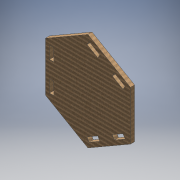
# Autodesk Inventor part: LightDiskTop
Saved by Autodesk Inventor 2016 (Build 200138000, 138)
## iProperties
Created: 2015-12-14
Part Number: LightDiskTop
Material: MDF Medium Density Fiberboard
Document SubType Name: Modeling
Designer: momem
Density: 0.8 g/cm^3
Appearance: Cardboard - Corrugated
Author: momem
Autodesk Inventor part; units mm, degrees
ref_plane "YZ Plane" through (0, 0, 0) normal (1, 0, 0) x (0, 1, 0)
ref_plane "XZ Plane" through (0, 0, 0) normal (0, 1, 0) x (-1, 0, 0)
ref_plane "XY Plane" through (0, 0, 0) normal (0, 0, 1) x (1, 0, 0)
sketch "Sketch1" plane through (0, 0, 0) normal (0, 1, 0) x (-1, 0, 0)
  circle A0 centre (0, 0) radius 30 construction
  line L0 (64.9519, -37.5) -> (0, -75)
  line L1 (0, -75) -> (-64.9519, -37.5)
  line L2 (-64.9519, -37.5) -> (-64.9519, 37.5)
  line L3 (-64.9519, 37.5) -> (0, 75)
  line L4 (0, 75) -> (64.9519, 37.5)
  line L5 (64.9519, 37.5) -> (64.9519, -37.5)
  line L6 (58.5619, 31.7388) -> (52.2358, 31.7388)
  line L7 (52.2358, 31.7388) -> (52.2358, 12.78)
  line L8 (52.2358, 12.78) -> (58.5619, 12.78)
  line L9 (58.5619, 12.78) -> (58.5619, 31.7388)
  line L10 (64.9519, 0) -> (0, 0) construction
  line L11 (58.5619, -31.7388) -> (52.2358, -31.7388)
  line L12 (52.2358, -31.7388) -> (52.2358, -12.78)
  line L13 (52.2358, -12.78) -> (58.5619, -12.78)
  line L14 (58.5619, -12.78) -> (58.5619, -31.7388)
  line L15 (-40.3488, 44.3261) -> (-56.7676, 34.8467)
  line L16 (-56.7676, 34.8467) -> (-53.6045, 29.3681)
  line L17 (-53.6045, 29.3681) -> (-37.1857, 38.8475)
  line L18 (-37.1857, 38.8475) -> (-40.3488, 44.3261)
  line L19 (-15.0501, 51.6275) -> (-18.2131, 57.1061)
  line L20 (-18.2131, 57.1061) -> (-1.7943, 66.5855)
  line L21 (-1.7943, 66.5855) -> (1.3687, 61.1069)
  line L22 (1.3687, 61.1069) -> (-15.0501, 51.6275)
  line L23 (-18.2131, -57.1061) -> (-1.7943, -66.5855)
  line L24 (-1.7943, -66.5855) -> (1.3687, -61.1069)
  line L25 (1.3687, -61.1069) -> (-15.0501, -51.6275)
  line L26 (-15.0501, -51.6275) -> (-18.2131, -57.1061)
  line L27 (-37.1857, -38.8475) -> (-40.3488, -44.3261)
  line L28 (-40.3488, -44.3261) -> (-56.7676, -34.8467)
  line L29 (-56.7676, -34.8467) -> (-53.6045, -29.3681)
  line L30 (-53.6045, -29.3681) -> (-37.1857, -38.8475)
  dimension "d0" = 60
  dimension "d2" = 150
  dimension "d3" = 6.3261
  dimension "d4" = 18.9588
  dimension "d5" = 6.39
  dimension "d6" = 12.78
  dimension "d9" = 360
  constraints: 62 end point, 4 symmetric about line, 2 coincident, 2 horizontal, 2 parallel, 1 centre point, 1 horizontal alignment, 1 midpoint, 1 perpendicular, 62 other
  measures "d0" diameter of A0
  measures "d2" distance of L2.end L0.start
  measures "d3" distance of L8.end L7.end
  measures "d4" distance of L6.end L7.end
  measures "d5" distance between parallel lines of L5 L9
  measures "d6" distance between parallel lines of L10 L8
extrude "Extrusion1" add sketch "Sketch1" along normal blind 6.39
equation "\"d3\" = 0.99 * WoodThickness"
equation "\"d4\" = 0.25 * DiskGap"
equation "\"d5\" = WoodThickness"
equation "\"d6\" = 2 * WoodThickness"
equation "\"d11\" = WoodThickness"
equation "\"WoodThickness\" = 6.39"
equation "\"DiskGap\" = 75.835317"
body "Solid1"
